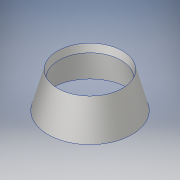
# Autodesk Inventor part: pheneolic_bottom
Saved by Autodesk Inventor 2017 SP1 (Build 210196100, 196)
## iProperties
Created: 2016-07-25
Part Number: pheneolic_bottom
Material: Aluminum 6061
Document SubType Name: Modeling
Designer: Jared
Density: 2.7 g/cm^3
Appearance: Aluminum - Flat
Author: Jared
Autodesk Inventor part; units mm, degrees
ref_plane "YZ Plane" through (0, 0, 0) normal (1, 0, 0) x (0, 1, 0)
ref_plane "XZ Plane" through (0, 0, 0) normal (0, 1, 0) x (-1, 0, 0)
ref_plane "XY Plane" through (0, 0, 0) normal (0, 0, 1) x (1, 0, 0)
sketch "Sketch1" plane through (0, 0, 0) normal (0, 0, 1) x (1, 0, 0)
  line L0 (0, 25.4) -> (-28.702, 25.4) construction
  line L1 (0, 25.4) -> (-95.25, 25.4) construction
  line L2 (-95.25, 25.4) -> (-92.075, 25.4) construction
  line L3 (-92.075, 25.4) -> (-85.725, 22.4389) construction
  line L4 (-92.075, 25.4) -> (-92.075, 22.4389) construction
  line L5 (-92.075, 0) -> (-95.25, 0)
  line L6 (-28.702, 59.6457) -> (-28.702, -91.9304) construction
  arc A0 (-28.9184, -9.8402) -> (-32.3684, -2.4417) centre (-35.052, -8.1967) ccw
  line L7 (-86.36, -224.2153) -> (-19.4758, 25.4)
  line L8 (-92.075, 25.4) -> (-92.075, 0)
  line L9 (-92.075, 25.4) -> (-32.3684, -2.4417)
  line L10 (-28.702, -9.0327) -> (-74.6859, -180.6468)
  line L11 (0, -319.0244) -> (0, 122.7573) projected
  line L12 (-73.152, 16.5761) -> (-52.4667, -97.7239)
  line L13 (-73.152, 16.5761) -> (-28.702, 16.5761) construction
  line L14 (-92.075, 0) -> (-95.25, 0)
  line L15 (-95.25, 0) -> (-95.25, -224.2153)
  line L16 (11.4547, -8.1967) -> (-136.2084, -8.1967) construction
  line L17 (-63.8887, -115.8166) -> (-82.55, -185.4617)
  line L18 (-95.25, -12.7) -> (-82.55, -12.7)
  line L19 (-82.55, -12.7) -> (-61.2385, -130.4605)
  line L20 (-95.25, -224.2153) -> (-86.36, -224.2153)
  line L21 (-82.55, -185.4617) -> (-75.976, -185.4617)
  point P0 (0, 0)
  point P1 (-95.25, -255.9127)
  point P2 (-88.7095, 22.4389)
  dimension "d0" = 28.702
  dimension "d3" = 25
  dimension "d5" = 25.4
  dimension "d6" = 25.4
  dimension "d8" = 12.7
  dimension "d34" = 15
  dimension "d37" = 44.45
  dimension "d38" = 114.3
  dimension "d40" = 95.25
  dimension "d41" = 3.175
  dimension "d46" = 12.7
  dimension "d47" = 12.7
  dimension "d50" = 86.36
  dimension "d51" = 12.7
  dimension "d52" = 6.35
  constraints: 42 end point, 19 point on line, 6 horizontal, 5 tangent, 3 perpendicular, 3 vertical, 2 parallel, 2 point on circle, 2 vertical alignment, 1 centre point, 1 coincident, 1 horizontal alignment
  measures "d0" distance of L0.start L0.end
  measures "d3" angle of L1 L3
  measures "d5" distance of point (0, 0) L0.start
  measures "d6" distance of L2.end L5.start
  measures "d8" diameter of A0
  measures "d34" angle of L6 L10
  measures "d37" distance of L12.start L13.end
  measures "d38" vertical distance of L12.start L12.end
  measures "d40" distance between parallel lines of L11 L15
  measures "d41" distance between parallel lines of L15 L8
  measures "d46" distance of L18.start L18.end
  measures "d47" distance between parallel lines of L14 L18
  measures "d50" distance from line of L11 L20.end
  measures "d51" distance from line of L15 L17.end
  measures "d52" distance between parallel lines of L7 L17
revolve "Revolution2" add sketch "Sketch1" angle 360 about axis through (0, -10, 0) along (0, 1, 0) contours L19 L7 L21 L17
body "Solid2"
